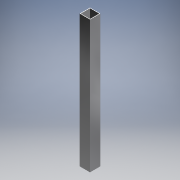
# Autodesk Inventor part: Convery frame2
Saved by Autodesk Inventor 2017 (Build 210142000, 142)
## iProperties
Created: 2020-02-21
Part Number: Convery frame2
Material: Aluminum 6061
Document SubType Name: Sheet Metal
Designer: S346553810
Density: 2.7 g/cm^3
Sheet Metal Rule: Default
Appearance: Aluminum - Flat
Author: S346553810
Autodesk Inventor part; units mm, degrees
ref_plane "YZ Plane" through (0, 0, 0) normal (1, 0, 0) x (0, 1, 0)
ref_plane "XZ Plane" through (0, 0, 0) normal (0, 1, 0) x (-1, 0, 0)
ref_plane "XY Plane" through (0, 0, 0) normal (0, 0, 1) x (1, 0, 0)
sketch "Sketch1" plane through (0, 0, 0) normal (0, 1, 0) x (-1, 0, 0)
  line L0 (-12.7, -12.7) -> (12.7, -12.7)
  line L1 (12.7, -12.7) -> (12.7, 12.7)
  line L2 (12.7, 12.7) -> (-12.7, 12.7)
  line L3 (-12.7, 12.7) -> (-12.7, -12.7)
  line L4 (-12.7, -12.7) -> (12.7, 12.7) construction
  line L5 (12.7, -12.7) -> (-12.7, 12.7) construction
  line L6 (-11.43, -11.43) -> (11.43, -11.43)
  line L7 (11.43, -11.43) -> (11.43, 11.43)
  line L8 (11.43, 11.43) -> (-11.43, 11.43)
  line L9 (-11.43, 11.43) -> (-11.43, -11.43)
  line L10 (-11.43, -11.43) -> (11.43, 11.43) construction
  line L11 (11.43, -11.43) -> (-11.43, 11.43) construction
  point P0 (0, 0)
  dimension "d0" = 25.4
  dimension "d1" = 25.4
  dimension "d2" = 22.86
  dimension "d3" = 22.86
  constraints: 24 end point, 4 midpoint, 4 parallel, 2 horizontal, 2 perpendicular
  measures "d0" distance of L2.end L1.end
  measures "d1" distance of L1.end L0.end
  measures "d2" distance of L8.end L7.end
  measures "d3" distance of L7.end L6.end
extrude "Extrusion1" add sketch "Sketch1" along normal blind 327.3044
sketch "Sketch2" plane through (0, 327.3044, 0) normal (0, 1, 0) x (1, 0, 0)
  line L0 (11.43, 11.43) -> (11.43, -11.43) projected
  line L1 (11.43, -11.43) -> (-11.43, -11.43) projected
  line L2 (-11.43, -11.43) -> (-11.43, 11.43) projected
  line L3 (-11.43, 11.43) -> (11.43, 11.43) projected
  line L4 (12.7, 12.7) -> (-12.7, 12.7) projected
  line L5 (-12.7, 12.7) -> (-12.7, -12.7) projected
  line L6 (-12.7, -12.7) -> (12.7, -12.7) projected
  line L7 (12.7, -12.7) -> (12.7, 12.7) projected
  point P0 (0, 0)
extrude "Extrusion2" add sketch "Sketch2" against normal blind 327.3044
sketch "Sketch5" plane through (12.7, 0, -12.7) normal (0, 0, -1) x (-1, 0, 0)
  circle A0 centre (12.7, 319.1401) radius 6.35
  line L0 (106.09, 453.881) -> (-174.2251, -6.5402) construction
  line L1 (78.7715, 457.8537) -> (-195.9205, 6.6684) construction
  line L2 (-0.7099, 327.3044) -> (20.9855, 314.0957) construction
  point P0 (12.7, 0)
  dimension "d12" = 12.7
  constraints: 3 point on line, 2 end point, 1 centre point, 1 perpendicular
  measures "d12" diameter of A0
extrude "Extrusion4" cut sketch "Sketch5" against normal blind 59.9694
equation "\"BendRadius\" = Thickness"
equation "\"BendReliefWidth\" = Thickness"
equation "\"BendReliefDepth\" = 0.5 * Thickness"
equation "\"CornerReliefSize\" = 4 * Thickness"
equation "\"MinimumRemnant\" = 2 * Thickness"
equation "\"TransitionRadius\" = BendRadius"
equation "\"JacobiRadiusSize\" = BendRadius"
equation "\"GapSize\" = Thickness"
equation "\"Thickness\" = 3.048"
body "Solid1"
